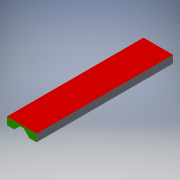
# Autodesk Inventor part: Holder_Slide_Top
Saved by Autodesk Inventor 2019 (Build 230136000, 136)
## iProperties
Created: 2021-01-21
Part Number: Holder_Slide_Top
Material: Generic
Document SubType Name: Modeling
Designer: zhanb
Density: 1 g/cm^3
Appearance: Default
Author: zhanb
Autodesk Inventor part; units mm, degrees
ref_plane "YZ Plane" through (0, 0, 0) normal (1, 0, 0) x (0, 1, 0)
ref_plane "XZ Plane" through (0, 0, 0) normal (0, 1, 0) x (-1, 0, 0)
ref_plane "XY Plane" through (0, 0, 0) normal (0, 0, 1) x (1, 0, 0)
sketch "Sketch1" plane through (0, 0, 0) normal (0, 1, 0) x (-1, 0, 0)
  line L0 (12.3825, 57.15) -> (-12.3825, 57.15)
  line L1 (-12.3825, 57.15) -> (-12.3825, -57.15)
  line L2 (-12.3825, -57.15) -> (12.3825, -57.15)
  line L3 (12.3825, -57.15) -> (12.3825, 57.15)
  line L4 (12.3825, 57.15) -> (-12.3825, -57.15) construction
  line L5 (-12.3825, 57.15) -> (12.3825, -57.15) construction
  point P0 (0, 0)
  dimension "d0" = 24.765
  dimension "d1" = 114.3
  constraints: 12 end point, 2 midpoint, 2 parallel, 1 horizontal, 1 perpendicular
  measures "d0" distance of L2.end L1.end
  measures "d1" distance of L1.end L0.end
extrude "Extrusion1" add sketch "Sketch1" along normal blind 6.35
sketch "Sketch2" plane through (-12.3825, 0, 57.15) normal (0, 0, 1) x (1, 0, 0)
  line L0 (6.096, 0) -> (18.669, 0)
  line L1 (0, 0) -> (24.765, 0) projected
  line L2 (18.669, 0) -> (13.97, 4.699)
  line L3 (13.97, 4.699) -> (10.795, 4.699)
  line L4 (10.795, 4.699) -> (6.096, 0)
  line L5 (0, 6.35) -> (24.765, 6.35) projected
  point P0 (12.3825, 0)
  point P1 (12.3825, 4.699)
  point P2 (12.3825, 6.35)
  dimension "d4" = 45
  dimension "d5" = 45
  dimension "d6" = 3.175
  dimension "d7" = 4.699
  constraints: 8 end point, 2 midpoint, 1 horizontal, 1 perpendicular, 1 point on line, 1 vertical alignment
  measures "d4" angle of L0 L4
  measures "d5" angle of L1 L2
  measures "d6" distance of L2.end L3.end
  measures "d7" vertical distance of L1.end L2.end
extrude "Extrusion2" cut sketch "Sketch2" against normal through all
sketch "Sketch3" plane through (0, 6.35, 0) normal (0, 1, 0) x (1, 0, 0)
  line L0 (12.3825, 57.15) -> (-12.3825, 57.15) construction
  line L1 (3.175, 57.15) -> (-3.175, 57.15)
  line L2 (-3.175, 57.15) -> (-3.175, 0)
  line L3 (3.175, 0) -> (3.175, 57.15)
  arc A0 (-3.175, 0) -> (3.175, 0) centre (0, 0) ccw
  dimension "d14" = 3.175
  dimension "d15" = 57.15
  constraints: 6 end point, 2 point on circle, 2 tangent, 1 centre point, 1 coincident, 1 horizontal, 1 parallel, 1 perpendicular, 1 point on line
  measures "d14" radius of A0
  measures "d15" distance from line of L0 A0.centre
extrude "Extrusion3" cut sketch "Sketch3" against normal through all
ref_plane "Work Plane1" through (12.3825, 0, -23.8125) normal (0, 0, -1) x (-1, 0, 0)
sketch "Sketch4" plane through (12.3825, 0, -23.8125) normal (0, 0, -1) x (-1, 0, 0)
  line L0 (9.2075, 3.1115) -> (9.2075, 6.35) construction
  line L1 (0, 6.35) -> (9.2075, 6.35) construction
  line L2 (0, 0) -> (0, 6.35) construction
  line L3 (0, 0) -> (6.096, 0) construction
  line L4 (6.096, 0) -> (9.2075, 3.1115) construction
  line L5 (0, 0) -> (6.096, 0) projected
  line L6 (1.016, 0) -> (0, 0)
  line L7 (0, 0) -> (0, 6.35)
  line L8 (0, 6.35) -> (9.2075, 6.35) projected
  line L9 (3.175, 6.35) -> (0, 6.35)
  line L10 (3.175, 6.35) -> (1.016, 5.1035)
  line L11 (1.016, 5.1035) -> (1.016, 0)
  point P0 (12.3825, 0)
  dimension "d19" = 150
  dimension "d20" = 1.016
  dimension "d21" = 3.175
  constraints: 10 end point, 2 collinear, 2 point on line, 1 parallel, 1 perpendicular
  measures "d19" angle of L1 L10
  measures "d20" distance between parallel lines of L2 L11
  measures "d21" distance of L1.start L9.start
extrude "Extrusion4" cut sketch "Sketch4" along normal mid plane 3.175
mirror "Mirror1" about plane through (0, 0, 0) normal (1, 0, 0) of "Extrusion4"
pattern_linear "Rectangular Pattern1" count 2 spacing 47.625 along (0, 0, 1) of "Extrusion4", "Mirror1"
sketch "Sketch6" plane through (-12.3825, 6.35, 57.15) normal (0, 0, 1) x (1, 0, 0)
  line L0 (6.096, -6.35) -> (10.795, -1.651) construction
  line L1 (10.795, -1.651) -> (13.97, -1.651) construction
  line L2 (13.97, -1.651) -> (18.669, -6.35) construction
  line L3 (18.669, -6.35) -> (24.765, -6.35) construction
  line L4 (24.765, -6.35) -> (24.765, 0) construction
  line L5 (0, 0) -> (24.765, 0) construction
  line L6 (0, -6.35) -> (0, 0) construction
  line L7 (0, -6.35) -> (6.096, -6.35) construction
  line L8 (9.2075, 0) -> (0, 0) projected
  line L9 (7.9559, 0) -> (9.4799, 1.524)
  line L10 (9.4799, 1.524) -> (15.2851, 1.524)
  line L11 (15.2851, 1.524) -> (16.8091, 0)
  line L12 (6.096, -6.35) -> (10.795, -1.651) projected
  line L13 (13.97, -1.651) -> (18.669, -6.35) projected
  line L14 (7.9559, 0) -> (16.8091, 0)
  line L15 (24.765, 0) -> (15.5575, 0) projected
  point P0 (12.3825, -6.35)
  point P1 (12.3825, 0)
  point P2 (12.3825, 1.524)
  dimension "d30" = 3.175
  dimension "d31" = 3.175
  constraints: 8 end point, 3 parallel, 2 midpoint, 2 point on line, 1 collinear, 1 vertical alignment
  measures "d30" distance between parallel lines of L10 L1
  measures "d31" distance between parallel lines of L2 L11
extrude "Extrusion5" add sketch "Sketch6" against normal blind 50.8
sketch "Sketch7" plane through (0, 6.35, 0) normal (0, 1, 0) x (1, 0, 0)
  line L0 (-9.2075, -22.225) -> (-9.2075, -25.4) projected
  line L1 (9.2075, -25.4) -> (9.2075, -22.225) projected
  line L2 (-9.2075, -25.4) -> (9.2075, -25.4)
  line L3 (9.2075, -25.4) -> (9.2075, -22.225)
  line L4 (9.2075, -22.225) -> (-9.2075, -22.225)
  line L5 (-9.2075, -22.225) -> (-9.2075, -25.4)
  point P0 (0, 0)
  constraints: 8 end point, 2 parallel, 1 horizontal, 1 perpendicular
extrude "Extrusion6" cut sketch "Sketch7" along normal through all
sketch "Sketch8" plane through (0, 6.35, 0) normal (0, 1, 0) x (1, 0, 0)
  line L0 (12.3825, -22.225) -> (11.3665, -22.225) construction
  line L1 (11.3665, -22.225) -> (11.3665, -25.4) construction
  line L2 (11.3665, -25.4) -> (12.3825, -25.4) construction
  line L3 (12.3825, -57.15) -> (12.3825, -25.4) construction
  line L4 (6.2865, -57.15) -> (12.3825, -57.15) construction
  line L5 (6.2865, -57.15) -> (6.2865, 57.15) construction
  line L6 (12.3825, 57.15) -> (6.2865, 57.15) construction
  line L7 (12.3825, 25.4) -> (12.3825, 57.15) construction
  line L8 (12.3825, 25.4) -> (11.3665, 25.4) construction
  line L9 (11.3665, 25.4) -> (11.3665, 22.225) construction
  line L10 (11.3665, 22.225) -> (12.3825, 22.225) construction
  line L11 (12.3825, -22.225) -> (12.3825, 22.225) construction
  line L12 (-11.3665, -22.225) -> (-12.3825, -22.225) construction
  line L13 (-12.3825, 22.225) -> (-12.3825, -22.225) construction
  line L14 (-12.3825, 22.225) -> (-11.3665, 22.225) construction
  line L15 (-11.3665, 22.225) -> (-11.3665, 25.4) construction
  line L16 (-11.3665, 25.4) -> (-12.3825, 25.4) construction
  line L17 (-12.3825, 57.15) -> (-12.3825, 25.4) construction
  line L18 (-6.2865, 57.15) -> (-12.3825, 57.15) construction
  line L19 (-6.2865, 57.15) -> (-6.2865, -57.15) construction
  line L20 (-12.3825, -57.15) -> (-6.2865, -57.15) construction
  line L21 (-12.3825, -25.4) -> (-12.3825, -57.15) construction
  line L22 (-12.3825, -25.4) -> (-11.3665, -25.4) construction
  line L23 (-11.3665, -25.4) -> (-11.3665, -22.225) construction
  line L24 (-12.3825, -25.4) -> (-12.3825, -57.15) projected
  line L25 (-12.3825, -28.575) -> (-9.3345, -31.623)
  line L26 (-9.3345, -31.623) -> (-9.3345, -57.15)
  line L27 (-12.3825, -57.15) -> (-6.2865, -57.15) projected
  line L28 (-12.3825, -57.15) -> (-9.3345, -57.15)
  line L29 (-12.3825, -57.15) -> (-12.3825, -28.575)
  line L30 (-12.3825, 57.15) -> (-12.3825, 25.4) construction
  line L31 (-12.3825, 28.575) -> (-9.525, 31.4325)
  line L32 (-9.525, 31.4325) -> (-3.175, 31.4325)
  line L33 (-3.175, 57.15) -> (-3.175, 0) construction
  line L34 (-3.175, 57.15) -> (-6.2865, 57.15) projected
  line L35 (-3.175, 31.4325) -> (-3.175, 57.15)
  line L36 (-3.175, 57.15) -> (-12.3825, 57.15)
  line L37 (-12.3825, 28.575) -> (-12.3825, 57.15)
  point P0 (0, 0)
  dimension "d36" = 45
  dimension "d37" = 3.175
  dimension "d38" = 3.175
  dimension "d39" = 45
  dimension "d40" = 6.35
  constraints: 18 end point, 3 point on line, 2 perpendicular, 2 vertical, 1 collinear, 1 horizontal, 1 midpoint, 1 parallel
  measures "d36" angle of L24 L25
  measures "d37" distance of L21.start L25.start
  measures "d38" distance of L16.end L31.start
  measures "d39" angle of L37 L31
  measures "d40" distance of L31.end L32.end
extrude "Extrusion7" cut sketch "Sketch8" against normal through all
mirror "Mirror2" about plane through (0, 0, 0) normal (1, 0, 0) of "Extrusion7"
equation "\"d38\" = d37"
equation "\"d39\" = d36"
body "Solid1"
